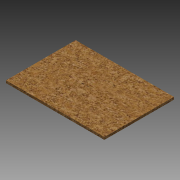
# Autodesk Inventor part: drzwiczki-bok
Saved by Autodesk Inventor 2013 (Build 170138000, 138)
## iProperties
Created: 2014-04-26
Part Number: drzwiczki-bok
Material: Generic
Document SubType Name: Modeling
Designer: Masta
Density: 1 g/cm^3
Author: Masta
Autodesk Inventor part; units mm, degrees
ref_plane "YZ Plane" through (0, 0, 0) normal (1, 0, 0) x (0, 1, 0)
ref_plane "XZ Plane" through (0, 0, 0) normal (0, 1, 0) x (-1, 0, 0)
ref_plane "XY Plane" through (0, 0, 0) normal (0, 0, 1) x (1, 0, 0)
sketch "Sketch1" plane through (0, 0, 0) normal (0, 0, 1) x (1, 0, 0)
  line L0 (-366, -259) -> (366, -259)
  line L1 (366, -259) -> (366, 259)
  line L2 (366, 259) -> (-366, 259)
  line L3 (-366, 259) -> (-366, -259)
  line L4 (-366, -259) -> (366, 259) construction
  line L5 (366, -259) -> (-366, 259) construction
  point P0 (0, 0)
  dimension "d0" = 732
  dimension "d1" = 518
  constraints: 12 end point, 2 midpoint, 2 parallel, 1 horizontal, 1 perpendicular
  measures "d0" distance of L2.end L1.end
  measures "d1" distance of L1.end L0.end
extrude "Extrusion1" add sketch "Sketch1" along normal blind 18
body "Solid1"
